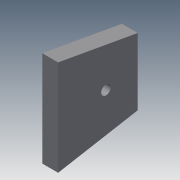
# Autodesk Inventor part: stojan_cast1
Saved by Autodesk Inventor 2013 (Build 170138000, 138)
## iProperties
Created: 2013-01-27
Part Number: stojan_cast1
Material: Generic
Document SubType Name: Modeling
Designer: idle-rug
Density: 1 g/cm^3
Author: idle-rug
Autodesk Inventor part; units mm, degrees
ref_plane "YZ Plane" through (0, 0, 0) normal (1, 0, 0) x (0, 1, 0)
ref_plane "XZ Plane" through (0, 0, 0) normal (0, 1, 0) x (-1, 0, 0)
ref_plane "XY Plane" through (0, 0, 0) normal (0, 0, 1) x (1, 0, 0)
sketch "Sketch1" plane through (0, 0, 0) normal (1, 0, 0) x (0, 1, 0)
  circle A0 centre (0, 0) radius 3
  line L0 (20, 0) -> (20, 21)
  line L1 (20, 0) -> (20, -21)
  line L2 (-30, 30) -> (-30, -30)
  line L3 (20, 21) -> (-30, 30)
  line L4 (20, -21) -> (-30, -30)
  constraints: 10 end point, 1 centre point, 1 coincident
extrude "Extrusion1" add sketch "Sketch1" along normal blind 10
body "Solid1"
